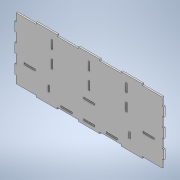
# Autodesk Inventor part: back
Saved by Autodesk Inventor 2020 (Build 240168000, 168)
## iProperties
Created: 2020-02-22
Part Number: back
Material: Generic
Document SubType Name: Modeling
Designer: udvarhelyi
Density: 1 g/cm^3
Appearance: Default
Author: udvarhelyi
Autodesk Inventor part; units mm, degrees
ref_plane "YZ Plane" through (0, 0, 0) normal (1, 0, 0) x (0, 1, 0)
ref_plane "XZ Plane" through (0, 0, 0) normal (0, 1, 0) x (-1, 0, 0)
ref_plane "XY Plane" through (0, 0, 0) normal (0, 0, 1) x (1, 0, 0)
sketch "Sketch1" plane through (0, 0, 0) normal (0, 0, 1) x (1, 0, 0)
  line L0 (-150, 18.5714) -> (-147, 18.5714)
  line L1 (-147, 37.1429) -> (-150, 37.1429)
  line L2 (-150, 55.7143) -> (-147, 55.7143)
  line L3 (-147, 74.2857) -> (-150, 74.2857)
  line L4 (-150, 92.8571) -> (-147, 92.8571)
  line L5 (-147, 111.4286) -> (-150, 111.4286)
  line L6 (147, 18.5714) -> (150, 18.5714)
  line L7 (147, 37.1429) -> (150, 37.1429)
  line L8 (150, 55.7143) -> (147, 55.7143)
  line L9 (147, 74.2857) -> (150, 74.2857)
  line L10 (150, 92.8571) -> (147, 92.8571)
  line L11 (150, 111.4286) -> (147, 111.4286)
  line L12 (-107.1429, 0) -> (-107.1429, 3)
  line L13 (-64.2857, 3) -> (-64.2857, 0)
  line L14 (-21.4286, 0) -> (-21.4286, 3)
  line L15 (21.4286, 0) -> (21.4286, 3)
  line L16 (64.2857, 0) -> (64.2857, 3)
  line L17 (107.1429, 0) -> (107.1429, 3)
  line L18 (-107.1429, 127) -> (-107.1429, 130)
  line L19 (-64.2857, 127) -> (-64.2857, 130)
  line L20 (-21.4286, 127) -> (-21.4286, 130)
  line L21 (21.4286, 127) -> (21.4286, 130)
  line L22 (64.2857, 127) -> (64.2857, 130)
  line L23 (107.1429, 127) -> (107.1429, 130)
  line L24 (-107.1429, 3) -> (-147, 3)
  line L25 (-147, 3) -> (-147, 18.5714)
  line L26 (-147, 37.1429) -> (-147, 55.7143)
  line L27 (-147, 74.2857) -> (-147, 92.8571)
  line L28 (-147, 111.4286) -> (-147, 127)
  line L29 (-147, 127) -> (-107.1429, 127)
  line L30 (-64.2857, 127) -> (-21.4286, 127)
  line L31 (21.4286, 127) -> (64.2857, 127)
  line L32 (107.1429, 127) -> (147, 127)
  line L33 (-21.4286, 3) -> (-64.2857, 3)
  line L34 (147, 3) -> (107.1429, 3)
  line L35 (64.2857, 3) -> (21.4286, 3)
  line L36 (-150, 92.8571) -> (-150, 111.4286)
  line L37 (-150, 18.5714) -> (-150, 37.1429)
  line L38 (-150, 55.7143) -> (-150, 74.2857)
  line L39 (-64.2857, 0) -> (-107.1429, 0)
  line L40 (107.1429, 0) -> (64.2857, 0)
  line L41 (21.4286, 0) -> (-21.4286, 0)
  line L42 (-107.1429, 130) -> (-64.2857, 130)
  line L43 (-21.4286, 130) -> (21.4286, 130)
  line L44 (64.2857, 130) -> (107.1429, 130)
  line L45 (150, 37.1429) -> (150, 18.5714)
  line L46 (150, 111.4286) -> (150, 92.8571)
  line L47 (150, 74.2857) -> (150, 55.7143)
  line L48 (147, 127) -> (147, 111.4286)
  line L49 (147, 92.8571) -> (147, 74.2857)
  line L50 (147, 55.7143) -> (147, 37.1429)
  line L51 (147, 18.5714) -> (147, 3)
  point P0 (0, 0)
  dimension "d1" = 300
  dimension "d5" = 42.8571
  dimension "d6" = 150
  dimension "d7" = 85.7143
  dimension "d8" = 128.5714
  dimension "d9" = 171.4286
  dimension "d10" = 214.2857
  dimension "d11" = 257.1429
  dimension "d12" = 130
  dimension "d13" = 18.5714
  dimension "d14" = 0
  dimension "d15" = 3
  dimension "d16" = 37.1429
  dimension "d17" = 55.7143
  dimension "d18" = 74.2857
  dimension "d19" = 92.8571
  dimension "d20" = 111.4286
  dimension "d21" = 124
  dimension "d22" = 3
  dimension "d23" = 3
  constraints: 104 end point, 79 perpendicular, 53 parallel, 21 collinear, 18 point on line, 3 horizontal
  measures "d1" distance of L5.end L11.start
  measures "d5" distance from line of L17.start L45
  measures "d6" distance from line of L46 point (0, 0)
  measures "d7" distance from line of L45 L16.start
  measures "d8" distance from line of L45 L15.end
  measures "d9" distance from line of L45 L14.start
  measures "d10" distance from line of L45 L13.end
  measures "d11" distance from line of L45 L12.start
  measures "d12" distance from line of L43 point (0, 0)
  measures "d13" distance from line of L0.start L39
  measures "d14" distance from line of point (0, 0) L39
  measures "d15" distance of L12.start L12.end
  measures "d16" distance from line of L39 L1.end
  measures "d17" distance from line of L39 L2.end
  measures "d18" distance from line of L39 L3.end
  measures "d19" distance from line of L39 L4.end
  measures "d20" distance from line of L39 L5.end
  measures "d21" distance between parallel lines of L24 L29
  measures "d22" distance of L11.start L11.end
  measures "d23" distance of L5.start L5.end
extrude "Extrusion1" add sketch "Sketch1" along normal blind 3
sketch "Sketch2" plane through (0, 0, 3) normal (0, 0, 1) x (1, 0, 0)
  line L0 (-108.5714, 45) -> (-131.4286, 45)
  line L1 (-131.4286, 45) -> (-131.4286, 48)
  line L2 (-131.4286, 48) -> (-108.5714, 48)
  line L3 (-108.5714, 48) -> (-108.5714, 45)
  line L4 (-11.4286, 45) -> (11.4286, 45)
  line L5 (11.4286, 45) -> (11.4286, 48)
  line L6 (11.4286, 48) -> (-11.4286, 48)
  line L7 (-11.4286, 48) -> (-11.4286, 45)
  line L8 (108.5714, 45) -> (131.4286, 45)
  line L9 (131.4286, 45) -> (131.4286, 48)
  line L10 (131.4286, 48) -> (108.5714, 48)
  line L11 (108.5714, 48) -> (108.5714, 45)
  line L12 (-21.4286, 0) -> (21.4286, 0) projected
  line L13 (-11.4286, 10) -> (11.4286, 10)
  line L14 (11.4286, 10) -> (11.4286, 7)
  line L15 (11.4286, 7) -> (-11.4286, 7)
  line L16 (-11.4286, 7) -> (-11.4286, 10)
  line L17 (34.2857, 7) -> (57.1429, 7)
  line L18 (57.1429, 7) -> (57.1429, 10)
  line L19 (57.1429, 10) -> (34.2857, 10)
  line L20 (34.2857, 10) -> (34.2857, 7)
  line L21 (-34.2857, 7) -> (-57.1429, 7)
  line L22 (-57.1429, 7) -> (-57.1429, 10)
  line L23 (-57.1429, 10) -> (-34.2857, 10)
  line L24 (-34.2857, 10) -> (-34.2857, 7)
  line L25 (-80, 21.6667) -> (-83, 21.6667)
  line L26 (-83, 21.6667) -> (-83, 33.3333)
  line L27 (-83, 33.3333) -> (-80, 33.3333)
  line L28 (-80, 33.3333) -> (-80, 21.6667)
  line L29 (80, 21.6667) -> (83, 21.6667)
  line L30 (83, 21.6667) -> (83, 33.3333)
  line L31 (83, 33.3333) -> (80, 33.3333)
  line L32 (80, 33.3333) -> (80, 21.6667)
  point P0 (0, 0)
  point P1 (-120, 45)
  point P2 (120, 45)
  dimension "d26" = 22.8571
  dimension "d27" = 48
  dimension "d28" = 3
  dimension "d29" = 120
  dimension "d30" = 120
  dimension "d31" = 11.4286
  dimension "d34" = 7
  dimension "d35" = 3
  dimension "d36" = 22.8571
  dimension "d37" = 22.8571
  dimension "d38" = 3
  dimension "d39" = 3
  dimension "d40" = 11.6667
  dimension "d41" = 11.6667
  dimension "d42" = 22.8571
  dimension "d43" = 22.8571
  constraints: 64 end point, 16 parallel, 9 point on line, 8 horizontal, 8 perpendicular, 5 equal length, 2 collinear, 2 midpoint
  measures "d26" distance of L4.start L4.end
  measures "d27" distance between parallel lines of L12 L6
  measures "d28" distance of L8.end L9.end
  measures "d29" horizontal distance of point (-120, 45) point (0, 0)
  measures "d30" horizontal distance of point (0, 0) point (120, 45)
  measures "d31" distance from line of L5 point (0, 0)
  measures "d34" distance between parallel lines of L12 L15
  measures "d35" distance of L15.end L13.start
  measures "d36" distance between parallel lines of L20 L14
  measures "d37" distance from line of L24 L15.end
  measures "d38" distance of L26.end L27.end
  measures "d39" distance of L30.end L31.end
  measures "d40" distance of L25.end L26.end
  measures "d41" distance between parallel lines of L23 L25
  measures "d42" distance between parallel lines of L22 L28
  measures "d43" distance between parallel lines of L32 L18
extrude "Extrusion2" cut sketch "Sketch2" against normal through all
sketch "Sketch3" plane through (0, 0, 3) normal (0, 0, 1) x (1, 0, 0)
  line L0 (-76.5, 116) -> (-73.5, 116)
  line L1 (-73.5, 116) -> (-73.5, 99)
  line L2 (-73.5, 99) -> (-76.5, 99)
  line L3 (-76.5, 99) -> (-76.5, 116)
  line L4 (-76.5, 82) -> (-73.5, 82)
  line L5 (-73.5, 82) -> (-73.5, 65)
  line L6 (-73.5, 65) -> (-76.5, 65)
  line L7 (-76.5, 65) -> (-76.5, 82)
  line L8 (-21.4286, 127) -> (-64.2857, 127) projected
  line L9 (-64.2857, 127) -> (-73.5, 127) construction
  line L10 (-73.5, 127) -> (-73.5, 116) construction
  line L11 (-73.5, 99) -> (-73.5, 82) construction
  line L12 (-108.5714, 48) -> (-73.5, 48) construction
  line L13 (-73.5, 48) -> (-73.5, 65) construction
  point P0 (0, 0)
  dimension "d44" = 17
  dimension "d45" = 3
  dimension "d46" = 73.5
  dimension "d52" = 17
  constraints: 26 end point, 4 horizontal, 4 parallel, 4 perpendicular, 3 collinear, 2 point on line
  measures "d44" distance of L2.end L0.start
  measures "d45" distance of L0.start L0.end
  measures "d46" distance from line of point (0, 0) L1
  measures "d52" distance of L1.end L4.end
extrude "Extrusion3" cut sketch "Sketch3" against normal through all
pattern_linear "Rectangular Pattern1" count 3 spacing 75 along (1, 0, 0) of "Extrusion3"
equation "\"d1\" = wt"
equation "\"d5\" = 0.142857 * wt - tol"
equation "\"d6\" = 0.5 * wt"
equation "\"d7\" = 0.285714 * wt + tol"
equation "\"d8\" = 0.428571 * wt - tol"
equation "\"d9\" = 0.571429 * wt + tol"
equation "\"d10\" = 0.714286 * wt - tol"
equation "\"d11\" = 0.857143 * wt + tol"
equation "\"d12\" = height_back"
equation "\"d13\" = 0.142857 * height_back - tol"
equation "\"d15\" = tt"
equation "\"d16\" = 0.285714 * height_back + tol"
equation "\"d17\" = 0.428571 * height_back - tol"
equation "\"d18\" = 0.571429 * height_back + tol"
equation "\"d19\" = 0.714286 * height_back - tol"
equation "\"d20\" = 0.857143 * height_back + tol"
equation "\"d21\" = -2 * tt + height_back"
equation "\"d22\" = tt"
equation "\"d23\" = tt"
equation "\"d24\" = tt"
equation "\"d26\" = 0.142857 * shelfW + 2 * tol"
equation "\"d28\" = tt"
equation "\"d29\" = 0.4 * wt"
equation "\"d30\" = 0.4 * wt"
equation "\"d31\" = 0.0714286 * shelfW + tol"
equation "\"d35\" = tt"
equation "\"d36\" = 0.142857 * shelfW - 2 * tol"
equation "\"d37\" = 0.142857 * shelfW - 2 * tol"
equation "\"d38\" = tt"
equation "\"d39\" = tt"
equation "\"d40\" = 0.333333 * shelfH + 2 * tol"
equation "\"d41\" = 0.333333 * shelfH - tol"
equation "\"d42\" = 0.142857 * shelfW - tol"
equation "\"d43\" = 0.142857 * shelfW - tol"
equation "\"d45\" = tt"
equation "\"d46\" = 0.25 * wt - 0.5 * tt"
equation "\"d51\" = 0.25 * wt"
equation "\"wt\" = 300"
equation "\"tt\" = 3"
equation "\"tol\" = 0"
equation "\"height_back\" = 130"
equation "\"d4\" = tt"
equation "\"tiroir\" = 1"
equation "\"nHoles\" = 4"
equation "\"shelfH\" = 35"
equation "\"shelfW\" = 160"
body "Solid1"
